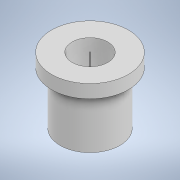
# Autodesk Inventor part: .25eyelet
Saved by Autodesk Inventor 2020 (Build 240168000, 168)
## iProperties
Created: 2019-06-20
Part Number: .25eyelet
Material: Generic
Document SubType Name: Modeling
Designer: ColinP
Density: 1 g/cm^3
Appearance: Default
Author: ColinP
Autodesk Inventor part; units mm, degrees
ref_plane "YZ Plane" through (0, 0, 0) normal (1, 0, 0) x (0, 1, 0)
ref_plane "XZ Plane" through (0, 0, 0) normal (0, 1, 0) x (-1, 0, 0)
ref_plane "XY Plane" through (0, 0, 0) normal (0, 0, 1) x (1, 0, 0)
sketch "Sketch2" plane through (0, 0, 0) normal (0, 0, 1) x (1, 0, 0)
  line L0 (0, 0) -> (0, 12.088)
  constraints: 2 end point, 1 vertical
sketch "Sketch3" plane through (0, 0, 0) normal (0, 0, 1) x (1, 0, 0)
  line L0 (0, 0) -> (5.4483, 0)
  line L1 (0, 0) -> (3.2512, 0)
  line L2 (3.2512, 0) -> (3.2512, 12.0142)
  line L3 (3.2512, 12.0142) -> (0, 12.0142)
  line L4 (0, 12.0142) -> (7.0104, 12.0142)
  line L5 (5.4483, 0) -> (5.4483, 9.6012)
  line L6 (5.4483, 9.6012) -> (7.0104, 9.6012)
  line L7 (7.0104, 9.6012) -> (7.0104, 12.0142)
  dimension "d8" = 5.4483
  dimension "d9" = 3.2512
  dimension "d10" = 12.0142
  dimension "d11" = 7.0104
  dimension "d12" = 9.6012
  constraints: 16 end point, 4 perpendicular, 2 point on line, 1 horizontal, 1 vertical
  measures "d8" distance of L0.start L0.end
  measures "d9" distance of L0.start L1.end
  measures "d10" distance of L1.end L2.end
  measures "d11" distance of L3.end L4.end
  measures "d12" distance of L0.end L5.end
revolve "Revolution1" add sketch "Sketch3" angle 360 about axis through (0, 0, 0) along (0, 1, 0)
body "Solid1"
